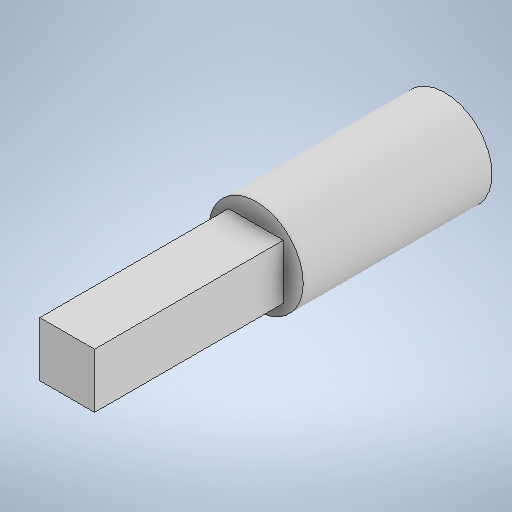
# Autodesk Inventor part: MINI Stepper Shaft ( Pinion )
Saved by Autodesk Inventor 2025.4 (Build 294407000, 407)
## iProperties
Created: 2026-04-11
Part Number: MINI Stepper Shaft ( Pinion )
Material: Generic
Document SubType Name: Modeling
Designer: lenovo
Density: 1 g/cm^3
Appearance: Default
Author: lenovo
Autodesk Inventor part; units mm, degrees
ref_plane "YZ Plane" through (0, 0, 0) normal (1, 0, 0) x (0, 1, 0)
ref_plane "XZ Plane" through (0, 0, 0) normal (0, 1, 0) x (-1, 0, 0)
ref_plane "XY Plane" through (0, 0, 0) normal (0, 0, 1) x (1, 0, 0)
sketch "Sketch1" plane through (0, 0, 0) normal (0, 0, 1) x (1, 0, 0)
  circle A0 centre (0, 0) radius 2.5
  dimension "d0" = 5
  constraints: 1 centre point, 1 coincident
  measures "d0" diameter of A0
extrude "Extrusion1" add sketch "Sketch1" along normal blind 10
sketch "Sketch2" plane through (0, 0, 10) normal (0, 0, 1) x (1, 0, 0)
  line L0 (-1.45, 1.45) -> (1.45, 1.45)
  line L1 (1.45, 1.45) -> (1.45, -1.45)
  line L2 (1.45, -1.45) -> (-1.45, -1.45)
  line L3 (-1.45, -1.45) -> (-1.45, 1.45)
  line L4 (-1.45, 1.45) -> (1.45, -1.45) construction
  line L5 (1.45, 1.45) -> (-1.45, -1.45) construction
  point P0 (0, 0)
  dimension "d3" = 2.9
  constraints: 12 end point, 2 midpoint, 2 parallel, 2 perpendicular, 1 horizontal
  measures "d3" distance of L0.end L1.end
extrude "Extrusion2" add sketch "Sketch2" along normal blind 10
body "Solid1"
